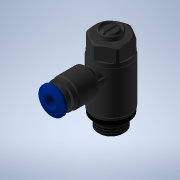
# Autodesk Inventor part: 193143 GRLA-1/8-QS-4-D
Saved by Autodesk Inventor 2021 (Build 250183000, 183)
## iProperties
Created: 2025-06-23
Part Number: 193143 GRLA-1/8-QS-4-D
Material: Generic
Catalog Web Link: www.cadenas.de
Description: GRLA-D-one-way flow control valve
Vendor: FESTO
Document SubType Name: Modeling
Designer: psAdmin
Manufacturer: FESTO
Mass: 22 g
Surface Area: 26.5243 cm^2
Volume: 4.67498 cm^3
Density: 1 g/cm^3
Appearance: PSOLRGB-175-175-175
Category: PARTsolutions
Company: FESTO
Title: 193143 GRLA-1/8-QS-4-D
Author: Cadenas PARTsolutions
Comments: one-way flow control valve
PSOL_IDENT_0: {$CADENAS_DATA/23d-libs/festo/parts/g/grla/grla_d.prj},184 {VTYP=3D},{NB=193143 GRLA-1/8-QS-4-D},{LI
PSOL_IDENT_1: NA=193143 GRLA-1/8-QS-4-D},{NN=GRLA-D},{DATE=02.05.2025 09:35:38},{GEOMDATE=20.03.2025 09:32:41},{VE
PSOL_IDENT_2: RSION=},{LINEID=50},{WBVAR=},{WBNUMERIC=}  {NB=193143 GRLA-1/8-QS-4-D},{LINA=193143 GRLA-1/8-QS-4-D}
PSOL_IDENT_3: ,{KT=DUMMY},{TNR=193143},{TYP=GRLA-1/8-QS-4-D},{INFO=},{FDTQS=-},{FDTQSV2=-},{FDTQS1=-},{FDTQS2=-},{
PSOL_IDENT_4: FDTQSDGST=-},{ZOLL=1/8},{VERS=1.000},{D=G1/8},{QS=QS-4},{ESTE=-},{DFC=-},{B=0.000},{DP=9.728},{KDRD=
PSOL_IDENT_5: 8.566},{D1=13.800},{D2=10.200},{DS=4.000},{H=29.400},{H1=22.500},{L=26.500},{L1=5.050},{L2=14.200},{
PSOL_IDENT_6: SW=12.000},{CNSMASSEXACT=0.02200},{MOM=3 ±0.3},{GB=1.600},{LHT=1.600},{TW=0.800},{DW=13.500},{DHT=7.
PSOL_IDENT_7: 500},{DCH=11.500},{DH=13.400},{HH=6.600},{HHB=8.100},{DI=3.000},{DIH=6.300},{LIH=0.530},{LTS=4.380},
PSOL_IDENT_8: {DSJ1=7.200},{DSJ2=8.200},{TSJ=3.000},{LSJ1=8.000},{LSJ2=18.600},{ASJ=45.000},{LSJ3=1.815},{LSJ4=0.0
PSOL_IDENT_9: 00},{LSJ5=3.100},{LSJ6=0.200},{DSJ3=4.200},{DSJ4=9.900},{DQS=0.000},{LQS=0.000},{DSJ5=7.500},{RSJ1=0
PSOL_IDENT_10: .200},{RSJ2=0.300},{DSJ6=5.400},{DSR=13.150},{TSR=1.600},{DSJ7=9.700},{HN=0.000},{DN=0.000},{DIN=0.0
PSOL_IDENT_11: 00},{DNC=0.000},{CHN=0.000},{RN=0.000},{HKH=0.000},{DKH=0.000},{DIKH=0.000},{DKHC=0.000},{CHKH=0.000
PSOL_IDENT_12: },{CHKH1=0.000},{RKH=0.000},{TKHS=0.000},{HSJ=0.000},{HSJN=0.000},{DAS=0.000},{TIH=1.520},{SRGH=0.30
PSOL_IDENT_13: 0},{DISR=12.150},{TQS=15.000},{EOLDATE=},{GTIN=4052568043834},{REACH=Ja},{REACHSVHC=Nein},{REACHHAZS
PSOL_IDENT_14: UBS=-},{REACHSCIP=-},{REACHVALDATE=-}
NB: 193143 GRLA-1/8-QS-4-D
NN: GRLA-D
NT: one-way flow control valve
NBSYN: $TNR. $TYP.
LINA: 193143 GRLA-1/8-QS-4-D
CATALOG: Festo
TNR: 193143
TYP: GRLA-1/8-QS-4-D
D: G1/8
QS: QS-4
ESTE: -
DFC: -
B: 0
D1: 13.8
D2: 10.2
DS: 4
H: 29.4
H1: 22.5
L: 26.5
L1: 5.05
L2: 14.2
SW: 12
CNSMASSEXACT: 0.022
MOM: 3 ±0.3
GTIN: 4052568043834
REACH: Yes
REACHSVHC: No
REACHHAZSUBS: -
REACHSCIP: -
REACHVALDATE: -
SUPPLIER: FESTO
ARTICLENO: 193143 GRLA-1/8-QS-4-D
BOMINFO: 193143 GRLA-1/8-QS-4-D
CREATOR: CADENAS GmbH
Autodesk Inventor part; units mm, degrees
sketch "Sketch_14" plane through (0, 0, 0) normal (1, 0, 0) x (0, 1, 0)
  line L0 (-19.25, 0) -> (12.3, 0)
  line L1 (12.3, 0) -> (12.3, -2.19)
  line L2 (12.3, -2.19) -> (10.7, -3.15)
  line L3 (10.7, -3.15) -> (11.77, -3.15)
  line L4 (11.77, -3.15) -> (12.3, -3.3971)
  line L5 (12.3, -3.3971) -> (12.3, -3.55)
  line L6 (12.3, -3.55) -> (12.1, -3.75)
  line L7 (12.1, -3.75) -> (10.7, -3.75)
  line L8 (10.7, -3.75) -> (10.7, -5.75)
  line L9 (10.7, -5.75) -> (10.1515, -6.7)
  line L10 (10.1515, -6.7) -> (4.2, -6.7)
  line L11 (4.2, -6.7) -> (4.2, -6.9)
  line L12 (4.2, -6.9) -> (-11.5, -6.9)
  line L13 (-11.5, -6.9) -> (-11.5, -6.075)
  arc A0 (-11.5, -6.075) -> (-11.8, -6.375) centre (-11.5, -6.375) ccw
  line L14 (-11.8, -6.375) -> (-11.8, -6.75)
  line L15 (-11.8, -6.75) -> (-12.6, -6.75)
  line L16 (-12.6, -6.75) -> (-12.6, -6.575)
  line L17 (-12.6, -6.575) -> (-14.2, -6.575)
  line L18 (-14.2, -6.575) -> (-14.2, -4.864)
  line L19 (-14.2, -4.864) -> (-18.669, -4.864)
  line L20 (-18.669, -4.864) -> (-19.25, -4.283)
  line L21 (-19.25, -4.283) -> (-19.25, 0)
  line L22 (-19.25, 0) -> (12.3, 0)
  constraints: 46 end point, 2 point on circle, 1 centre point
revolve "Revolution1" add sketch "Sketch_14" angle 360 about axis through (0, -19.25, 0) along (0, -1, 0)
thread "Thread1" size "G9.728x0.907" designation "G 1/8" class "A" standard "ISO Pipe Threads" full length
sketch "Sketch_15" plane through (0, 12.3, 0) normal (0, 1, 0) x (1, 0, 0)
  line L0 (-12, -6.9282) -> (0, -13.8564)
  line L1 (0, -13.8564) -> (12, -6.9282)
  line L2 (12, -6.9282) -> (12, 6.9282)
  line L3 (12, 6.9282) -> (0, 13.8564)
  line L4 (0, 13.8564) -> (-12, 6.9282)
  line L5 (-12, 6.9282) -> (-12, -6.9282)
  line L6 (-6, -3.4641) -> (0, -6.9282)
  line L7 (0, -6.9282) -> (6, -3.4641)
  line L8 (6, -3.4641) -> (6, 3.4641)
  line L9 (6, 3.4641) -> (0, 6.9282)
  line L10 (0, 6.9282) -> (-6, 3.4641)
  line L11 (-6, 3.4641) -> (-6, -3.4641)
  constraints: 24 end point
extrude "Extrusion1" cut sketch "Sketch_15" against normal blind 6.6
sketch "Sketch_16" plane through (0, 12.3, 0) normal (0, 1, 0) x (1, 0, 0)
  line L0 (-0.4, 3.0237) -> (-0.4, -3.0237)
  arc A0 (-0.4, -3.0237) -> (0.4, -3.0237) centre (0, 0) ccw
  line L1 (0.4, -3.0237) -> (0.4, 3.0237)
  arc A1 (0.4, 3.0237) -> (-0.4, 3.0237) centre (0, 0) ccw
  constraints: 4 end point, 4 point on circle, 2 centre point
extrude "Extrusion2" cut sketch "Sketch_16" against normal blind 1.2
sketch "Sketch_11" plane through (0, 0, 0) normal (1, 0, 0) x (0, 1, 0)
  line L0 (0, 0) -> (0, 22.5)
  line L1 (0, 22.5) -> (2.3, 22.5)
  line L2 (2.3, 22.5) -> (4.7847, 22.0619)
  arc A0 (4.95, 21.8649) -> (4.7847, 22.0619) centre (4.75, 21.8649) ccw
  line L3 (4.95, 21.8649) -> (4.95, 21)
  line L4 (4.95, 21) -> (3.1, 21)
  arc A1 (3.1, 21) -> (2.7, 20.6) centre (3.1, 20.6) ccw
  line L5 (2.7, 20.6) -> (2.7, 20)
  line L6 (2.7, 20) -> (3.55, 20)
  line L7 (3.55, 20) -> (3.75, 19.8)
  line L8 (3.75, 19.8) -> (3.75, 18.6)
  line L9 (3.75, 18.6) -> (4.85, 18.6)
  line L10 (4.85, 18.6) -> (4.85, 17.1)
  line L11 (4.85, 17.1) -> (5.1, 16.667)
  line L12 (5.1, 16.667) -> (5.1, 9.5)
  line L13 (5.1, 9.5) -> (3.6, 8)
  line L14 (3.6, 8) -> (3.6, 0)
  line L15 (3.6, 0) -> (0, 0)
  line L16 (0, 0) -> (0, 22.5)
  constraints: 34 end point, 4 point on circle, 2 centre point
revolve "Revolution2" add sketch "Sketch_11" angle 360 about axis through (0, 0, 0) along (0, 0, -1)
sketch "Sketch_17" plane through (0, 0, 0) normal (1, 0, 0) x (0, 1, 0)
  line L0 (0, 0) -> (0, 22.5)
  line L1 (0, 22.5) -> (2.3, 22.5)
  line L2 (2.3, 22.5) -> (4.7847, 22.0619)
  arc A0 (4.95, 21.8649) -> (4.7847, 22.0619) centre (4.75, 21.8649) ccw
  line L3 (4.95, 21.8649) -> (4.95, 21)
  line L4 (4.95, 21) -> (3.1, 21)
  arc A1 (3.1, 21) -> (2.7, 20.6) centre (3.1, 20.6) ccw
  line L5 (2.7, 20.6) -> (2.7, 20.085)
  line L6 (2.7, 20.085) -> (3.55, 20.085)
  line L7 (3.55, 20.085) -> (3.75, 19.885)
  line L8 (3.75, 19.885) -> (3.75, 18.6)
  line L9 (3.75, 18.6) -> (4.85, 18.6)
  line L10 (4.85, 18.6) -> (4.85, 17.1)
  line L11 (4.85, 17.1) -> (5.1, 16.667)
  line L12 (5.1, 16.667) -> (5.1, 9.5)
  line L13 (5.1, 9.5) -> (3.6, 8)
  line L14 (3.6, 8) -> (3.6, 0)
  line L15 (3.6, 0) -> (0, 0)
  line L16 (0, 0) -> (0, 22.5)
  constraints: 34 end point, 4 point on circle, 2 centre point
revolve "Revolution3" add sketch "Sketch_17" angle 360 about axis through (0, 0, 0) along (0, 0, -1)
sketch "Sketch_18" plane through (0, 0, 0) normal (0, 0, 1) x (1, 0, 0)
  arc A0 (-3.8158, 1.5) -> (-3.8158, -1.5) centre (0, 0) ccw
  line L0 (-3.8158, -1.5) -> (3.8158, -1.5)
  arc A1 (3.8158, -1.5) -> (3.8158, 1.5) centre (0, 0) ccw
  line L1 (3.8158, 1.5) -> (-3.8158, 1.5)
  constraints: 4 end point, 4 point on circle, 2 centre point
extrude "Extrusion3" add sketch "Sketch_18" along normal blind 11.25
sketch "Sketch_5" plane through (0, 0, 0) normal (1, 0, 0) x (0, 1, 0)
  line L0 (0, 0) -> (0, 22.5)
  line L1 (0, 22.5) -> (2.3, 22.5)
  arc A0 (2.3, 22.5) -> (2, 22.2) centre (2.3, 22.2) ccw
  line L2 (2, 22.2) -> (2, 7.5)
  line L3 (2, 7.5) -> (1, 7.5)
  line L4 (1, 7.5) -> (1, 0)
  line L5 (1, 0) -> (0, 0)
  line L6 (0, 0) -> (0, 22.5)
  constraints: 14 end point, 2 point on circle, 1 centre point
revolve "Revolution4" cut sketch "Sketch_5" angle 360 about axis through (0, 0, 0) along (0, 0, -1)
sketch "Sketch8" plane through (0, -19.25, 0) normal (0, -1, 0) x (1, 0, 0)
  point P0 (0, 0)
hole "Hole1" at (0, -19.25, 0) direction (0, 1, 0) diameter 3 depth 21.25 countersink diameter 3.3464 countersink angle 60
ref_plane "FDT_MOUNT_XY" through (0, -14.2, 0) normal (0, 1, 0) x (-1, 0, 0)
ref_plane "FDT_MOUNT_YZ" through (0, -14.2, 0) normal (-1, 0, 0) x (0, 0, 1)
ref_plane "FDT_MOUNT_ZX" through (0, -14.2, 0) normal (0, 0, 1) x (0, 1, 0)
ref_plane "FDT_SCHLAUCH_XY" through (0, 0, 7.5) normal (0, 0, 1) x (1, 0, 0)
ref_plane "FDT_SCHLAUCH_YZ" through (0, 0, 7.5) normal (1, 0, 0) x (0, 1, 0)
ref_plane "FDT_SCHLAUCH_ZX" through (0, 0, 7.5) normal (0, 1, 0) x (0, 0, 1)
ref_plane "Zylinder_XY" through (0, -19.25, 0) normal (0, 1, 0) x (1, 0, 0)
ref_plane "Zylinder_YZ" through (0, -19.25, 0) normal (1, 0, 0) x (0, 0, -1)
ref_plane "Zylinder_ZX" through (0, -19.25, 0) normal (0, 0, -1) x (0, 1, 0)
ref_plane "anbau_XY" through (0, -14.2, 0) normal (0, 1, 0) x (1, 0, 0)
ref_plane "anbau_YZ" through (0, -14.2, 0) normal (1, 0, 0) x (0, 0, -1)
ref_plane "anbau_ZX" through (0, -14.2, 0) normal (0, 0, -1) x (0, 1, 0)
body "Solid1"
